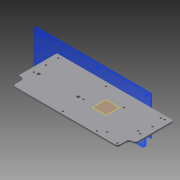
# Autodesk Inventor part: bakplate
Saved by Autodesk Inventor 2015 (Build 190159000, 159)
## iProperties
Created: 2015-07-23
Part Number: bakplate
Material: Generic
Document SubType Name: Modeling
Designer: Simen
Density: 1 g/cm^3
Appearance: Default
Author: Simen
Autodesk Inventor part; units mm, degrees
ref_plane "YZ Plane" through (0, 0, 0) normal (1, 0, 0) x (0, 1, 0)
ref_plane "XZ Plane" through (0, 0, 0) normal (0, 1, 0) x (-1, 0, 0)
ref_plane "XY Plane" through (0, 0, 0) normal (0, 0, 1) x (1, 0, 0)
ref_plane "Work Plane1" through (0, 0, 2.5) normal (0, 0, 1) x (1, 0, 0)
ref_plane "Work Plane2" through (0.1403, 1, -35.0827) normal (0, 0, 1) x (1, 0, 0)
sketch "Sketch3" plane through (0.1403, 1, -35.0827) normal (0, 0, 1) x (1, 0, 0)
  circle A0 centre (30.3585, 25) radius 1.5 projected
  circle A1 centre (30.3585, 45) radius 1.5 projected
  circle A2 centre (22.8585, 0) radius 1.5 projected
  circle A3 centre (-144.6415, 25) radius 1.5 projected
  circle A4 centre (-137.1415, 0) radius 1.5 projected
  circle A5 centre (-144.6415, 45) radius 1.5 projected
  circle A6 centre (-137.1415, 90) radius 1.5 projected
  circle A7 centre (-144.6415, 65) radius 1.5 projected
  circle A8 centre (0.8585, 0) radius 1.5 projected
  circle A9 centre (30.3585, 65) radius 1.5 projected
  circle A10 centre (22.8585, 90) radius 1.5 projected
  arc A11 (-148.6415, 82.5) -> (-153.6415, 77.5) centre (-148.6415, 77.5) ccw projected
  line L0 (-153.6415, 77.5) -> (-153.6415, 12.5) projected
  arc A12 (-153.6415, 12.5) -> (-148.6415, 7.5) centre (-148.6415, 12.5) ccw projected
  arc A13 (-143.6415, 2.5) -> (-148.6415, 7.5) centre (-148.6415, 2.5) ccw projected
  line L1 (-143.6415, 2.5) -> (-143.6415, -6.5) projected
  arc A14 (-143.6415, -6.5) -> (-138.6415, -11.5) centre (-138.6415, -6.5) ccw projected
  line L2 (-138.6415, -11.5) -> (24.3585, -11.5) projected
  arc A15 (24.3585, -11.5) -> (29.3585, -6.5) centre (24.3585, -6.5) ccw projected
  line L3 (29.3585, -6.5) -> (29.3585, 2.5) projected
  arc A16 (34.3585, 7.5) -> (29.3585, 2.5) centre (34.3585, 2.5) ccw projected
  arc A17 (34.3585, 7.5) -> (39.3585, 12.5) centre (34.3585, 12.5) ccw projected
  line L4 (39.3585, 12.5) -> (39.3585, 77.5) projected
  arc A18 (39.3585, 77.5) -> (34.3585, 82.5) centre (34.3585, 77.5) ccw projected
  arc A19 (29.3585, 87.5) -> (34.3585, 82.5) centre (34.3585, 87.5) ccw projected
  line L5 (29.3585, 87.5) -> (29.3585, 96.5) projected
  arc A20 (29.3585, 96.5) -> (24.3585, 101.5) centre (24.3585, 96.5) ccw projected
  line L6 (24.3585, 101.5) -> (-138.6415, 101.5) projected
  arc A21 (-138.6415, 101.5) -> (-143.6415, 96.5) centre (-138.6415, 96.5) ccw projected
  line L7 (-143.6415, 96.5) -> (-143.6415, 87.5) projected
  arc A22 (-148.6415, 82.5) -> (-143.6415, 87.5) centre (-148.6415, 87.5) ccw projected
  arc A23 (36.857, 12.4115) -> (36.8585, 12.5) centre (34.3585, 12.5) ccw
  line L8 (-152.6415, 8.382) -> (-152.6415, 9.5)
  line L9 (-95.0914, -11.5) -> (-95.0914, 101.5)
  arc A24 (37.5224, 9.3) -> (37.8585, 9.6716) centre (34.3585, 12.5) ccw
  line L10 (-152.6415, 12.5) -> (-152.6415, 64.5)
  line L11 (38.3585, 64.5) -> (38.3585, 12.5)
  arc A25 (34.3585, 8.5) -> (38.3585, 12.5) centre (34.3585, 12.5) ccw
  arc A26 (34.3585, 8.5) -> (28.3585, 2.5) centre (34.3585, 2.5) ccw
  line L12 (28.3585, 2.5) -> (28.3585, -6.5)
  arc A27 (24.3585, -10.5) -> (28.3585, -6.5) centre (24.3585, -6.5) ccw
  line L13 (24.3585, -10.5) -> (-138.6415, -10.5)
  arc A28 (-142.6415, -6.5) -> (-138.6415, -10.5) centre (-138.6415, -6.5) ccw
  line L14 (-142.6415, -6.5) -> (-142.6415, 2.5)
  arc A29 (-142.6415, 2.5) -> (-148.6415, 8.5) centre (-148.6415, 2.5) ccw
  arc A30 (-152.6415, 12.5) -> (-148.6415, 8.5) centre (-148.6415, 12.5) ccw
  line L15 (-57.1415, -10.5) -> (-57.1415, 69.5)
  line L16 (-57.1415, 69.5) -> (33.3585, 69.5)
  line L17 (-57.1415, 69.5) -> (-147.6415, 69.5)
  arc A31 (38.3585, 64.5) -> (33.3585, 69.5) centre (33.3585, 64.5) ccw
  arc A32 (-147.6415, 69.5) -> (-152.6415, 64.5) centre (-147.6415, 64.5) ccw
  point P0 (-0.1403, -1)
  point P1 (-151.6415, 9.5)
  point P2 (-152.6415, 69.5)
  dimension "d26" = 1
  dimension "d32" = 1
  dimension "d33" = 80
  dimension "d35" = 5
  constraints: 21 point on circle, 20 end point, 10 centre point, 5 point on line, 4 tangent, 2 perpendicular, 1 equal radius, 1 midpoint, 1 vertical, 9 other
  measures "d26" distance between parallel lines of L0 L8
  measures "d32" distance between parallel lines of L0 L10
  measures "d33" distance of L15.start L15.end
  measures "d35" radius of A31
extrude "Extrusion3" add sketch "Sketch3" along normal blind 2.5 contours A2 | L17 L15 L13 L9 | L9 L13 A28 L14 A29 A30 L10 A32 L17 | L16 A31 L11 A25 A26 L12 A27 L13 L15
sketch "Sketch5" plane through (0.1403, 1, -32.5827) normal (0, 0, 1) x (1, 0, 0)
  circle A0 centre (-137.6415, 27) radius 2.5 projected
  circle A1 centre (-72.6415, 27) radius 2.5 projected
  circle A2 centre (-144.6415, 65) radius 1.5 projected
  circle A3 centre (-144.6415, 45) radius 1.5 projected
  circle A4 centre (-144.6415, 25) radius 1.5 projected
  circle A5 centre (30.3585, 65) radius 1.5 projected
  circle A6 centre (0.8585, 0) radius 1.5 projected
  circle A7 centre (30.3585, 45) radius 1.5 projected
  circle A8 centre (30.3585, 25) radius 1.5 projected
  circle A9 centre (24.3585, -6.5) radius 1.5 projected
  circle A10 centre (-9.6415, -6.5) radius 1.5 projected
  circle A11 centre (24.3585, 27.5) radius 1.5 projected
  circle A12 centre (-65.6415, 27.5) radius 1.5 projected
  circle A13 centre (-65.6415, -6.5) radius 1.5 projected
  circle A14 centre (-65.6415, 64.5) radius 1.5 projected
  circle A15 centre (-20.6415, 49.5) radius 1.5 projected
  circle A16 centre (24.3585, 64.5) radius 1.5 projected
  point P0 (-0.1403, -1)
extrude "Extrusion6" cut sketch "Sketch5" against normal blind 10 contours A0 | A1 | A9 | A10 | A11 | A12 | A13 | A14 | A15 | A16
body "Solid3"
